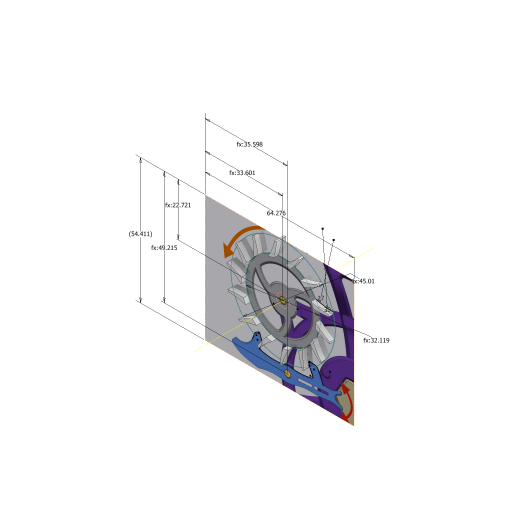
# Autodesk Inventor part: escapement
Saved by Autodesk Inventor 2023 (Build 270158000, 158)
## iProperties
Created: 2023-02-13
Part Number: escapement
Material: Generic
Document SubType Name: Modeling
Designer: me
Density: 1 g/cm^3
Appearance: Default
Author: me
Autodesk Inventor part; units mm, degrees
ref_plane "YZ Plane" through (0, 0, 0) normal (1, 0, 0) x (0, 1, 0)
ref_plane "XZ Plane" through (0, 0, 0) normal (0, 1, 0) x (-1, 0, 0)
sketch "Sketch1" plane through (0, 0, 0) normal (0, 0, 1) x (1, 0, 0)
  line L0 (0, 0) -> (64.2761, 0) construction
  line L1 (64.2761, 0) -> (64.2761, -54.4112) construction
  line L2 (64.2761, -54.4112) -> (0, -54.4112) construction
  line L3 (0, -54.4112) -> (0, 0) construction
  circle A0 centre (33.6015, -22.7208) radius 16.0597
  circle A1 centre (33.6015, -22.7208) radius 2.7704 construction
  circle A2 centre (33.6015, -22.7208) radius 22.505
  arc A3 (47.7163, -15.0601) -> (55.1406, -16.1985) centre (55.4809, 10.7994) ccw
  arc A4 (48.7, -17.2482) -> (55.3543, -16.951) centre (50.6967, 12.6853) ccw
  circle A5 centre (35.5981, -49.2149) radius 1.0018 construction
  line L4 (51.0158, -45.7993) -> (48.8436, -40.9549)
  line L5 (47.3838, -39.8895) -> (45.109, -39.6344)
  line L6 (46.331, -44.4438) -> (44.9184, -41.4816)
  arc A6 (48.8436, -40.9549) -> (47.3838, -39.8895) centre (47.1807, -41.7006) ccw
  arc A7 (45.109, -39.6344) -> (44.6585, -40.0822) centre (45.0636, -40.0392) ccw
  arc A8 (44.6585, -40.0822) -> (44.9031, -41.4393) centre (54.1179, -39.0783) ccw
  arc A9 (44.9031, -41.4393) -> (44.9184, -41.4816) centre (45.128, -41.3816) ccw
  line L7 (23.4876, -45.494) -> (24.3879, -43.6304)
  line L8 (24.4629, -42.2262) -> (23.6119, -39.8454)
  line L9 (23.1057, -39.6691) -> (21.763, -40.5062)
  line L10 (21.3843, -40.9575) -> (20.3787, -43.4532)
  arc A10 (24.3879, -43.6304) -> (24.4629, -42.2262) centre (22.7492, -42.8388) ccw
  arc A11 (23.6119, -39.8454) -> (23.1057, -39.6691) centre (23.2878, -39.9612) ccw
  arc A12 (21.763, -40.5062) -> (21.3843, -40.9575) centre (22.2659, -41.3128) ccw
  arc A13 (45.8085, -45.5494) -> (46.331, -44.4438) centre (45.6187, -44.7835) ccw
  arc A14 (35.8429, -45.8507) -> (45.8085, -45.5494) centre (40.1278, -22.6181) ccw
  arc A15 (23.651, -45.8667) -> (35.8429, -45.8507) centre (29.7207, -25.8248) ccw
  arc A16 (23.4876, -45.494) -> (23.651, -45.8667) centre (23.7286, -45.6105) ccw
  dimension "d10" = 64.2761
  dimension "d12" = 33.6015
  dimension "d14" = 54.4112
  dimension "d16" = 22.7208
  dimension "d46" = 45.01
  dimension "d49" = 32.1195
  dimension "d92" = 27
  dimension "d102" = 30
  dimension "d115" = 35.5981
  dimension "d116" = 49.2149
  constraints: 30 point on circle, 17 centre point, 16 tangent, 14 end point, 2 coincident, 1 horizontal, 4 other
  measures "d10" distance of L0.start L0.end
  measures "d12" distance from line of L3 A0.centre
  measures "d14" distance of L2.end L0.start
  measures "d16" vertical distance of L0.start A0.centre
  measures "d46" diameter of A2
  measures "d49" diameter of A0
  measures "d92" radius of A3
  measures "d102" radius of A4
  measures "d115" horizontal distance of L0.start A5.centre
  measures "d116" vertical distance of L0.start A5.centre
extrude "Extrusion1" add sketch "Sketch1" along normal mid plane 4 contours A0 A3 A2 A4
pattern_circular "Circular Pattern1" count 14 over 360 about axis through (33.6015, -22.7208, 0) along (0, 0, 1) of "Extrusion1"
equation "\"d12\" = 0.522768 * d10"
equation "\"d16\" = 0.417576 * d14"
equation "\"d46\" = 1.40133 * d49"
equation "\"d49\" = 0.499711 * d10"
equation "\"d115\" = 0.553832 * d10"
equation "\"d116\" = 0.9045 * d14"
